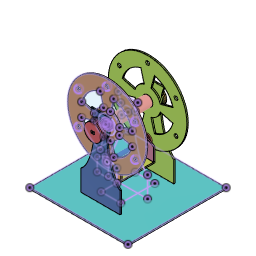
Ferris Wheel (Autodesk Fusion 360 design; units mm, degrees)
Autodesk Fusion 360 part; units mm, degrees
note: some values were not read from the file. Chosen so that the rebuilt part matches the saved one: where a step ends. Set by a fixed rule: which sketch regions a step uses.
sketch "01_base" plane through (0, 0, 0) normal (0, 0, 1) x (1, 0, 0) in component "05_centre_shaft"
  line L0 (75, -75) -> (-75, -75)
  line L1 (-75, -75) -> (-75, 75)
  line L2 (-75, 75) -> (75, 75)
  line L3 (75, 75) -> (75, -75)
  line L4 (75, -75) -> (-75, 75) construction
  line L5 (-75, -75) -> (75, 75) construction
  dimension "d1" = 150
  constraint horizontal L0
  constraint perpendicular L0 L1
  constraint parallel L0 L2
  constraint parallel L1 L3
  constraint coincident L4 origin
  constraint coincident L5 origin
  constraint equal L1 L2
  measures "d1" distance of L1.end L2.end
extrude "Extrude1" add sketch "01_base" along normal blind 2 makes body 1 in component "01_baseplate"
sketch "02_wheel" plane through (0, 0, 0) normal (0, 1, 0) x (1, 0, 0) in component "05_centre_shaft"
  circle A0 centre (0, -102) radius 60
  line L0 (-75, -2) -> (75, -2)
  line L1 (0, -1.75) -> (0, -22.5)
  circle A1 centre (0, -102) radius 40
  circle A2 centre (0, -152) radius 2.85
  line L2 (0, -162) -> (0, -142) construction
  circle A3 centre (43.3013, -127) radius 2.85
  circle A4 centre (43.3013, -77) radius 2.85
  circle A5 centre (0, -52) radius 2.85
  circle A6 centre (-43.3013, -77) radius 2.85
  circle A7 centre (-43.3013, -127) radius 2.85
  circle A8 centre (0, -102) radius 20
  line L3 (5.1764, -121.3185) -> (10.3528, -140.637)
  line L4 (-5.1764, -121.3185) -> (-10.3528, -140.637)
  line L5 (19.3185, -96.8236) -> (38.637, -91.6472)
  line L6 (19.3185, -107.1764) -> (38.637, -112.3528)
  line L7 (-5.1764, -82.6815) -> (-10.3528, -63.363)
  line L8 (5.1764, -82.6815) -> (10.3528, -63.363)
  line L9 (-19.3185, -107.1764) -> (-38.637, -112.3528)
  line L10 (-19.3185, -96.8236) -> (-38.637, -91.6472)
  circle A9 centre (0, -102) radius 7.95
  circle A10 centre (0, -52) radius 7
  line L11 (-3.5, -58.0622) -> (-15, -51.4226)
  line L12 (0, -42.7624) -> (0, -42)
  line L13 (0, -31.4226) -> (-15, -31.4226)
  line L14 (-15, -31.4226) -> (-15, -51.4226)
  line L15 (3.5, -58.0622) -> (15, -51.4226)
  line L16 (15, -31.4226) -> (15, -51.4226)
  line L17 (0, -31.4226) -> (15, -31.4226)
  point P0 (0, -152)
  dimension "d10" = 100
  dimension "d11" = 120
  dimension "d12" = -20
  dimension "d14" = 5.7
  dimension "d16" = 360
  dimension "d17" = -40
  dimension "d18" = 15
  dimension "d20" = 360
  dimension "d27" = 14
  dimension "d31" = 60
  dimension "d32" = 20
  dimension "d33" = 15
  dimension "d39" = 15.9
  constraint coincident A0.centre L1
  constraint coincident A0 L2.start
  constraint coincident A1 L2.end
  constraint coincident L1 L2.end
  constraint vertical L2
  constraint midpoint L2 P0
  constraint coincident P0 A2.centre
  constraint coincident A1 L3.end
  constraint coincident A8 L3.start
  constraint coincident A0.centre L3
  constraint symmetric L1 L3.end L4.end
  constraint symmetric L1 L3.start L4.start
  constraint concentric A0 A9
  constraint concentric A5 A10
  constraint tangent A10 L11
  constraint coincident A10 L11.start
  constraint vertical L12
  constraint horizontal L13
  constraint vertical L14
  constraint coincident L1 L13.start
  constraint coincident A0 L12.end
  constraint symmetric L1 L11.start L15.start
  constraint symmetric L1 L11.end L15.end
  constraint symmetric L1 L13.start L17.start
  constraint symmetric L1 L13.end L16.start
  measures "d10" distance of A0.centre L0
  measures "d11" diameter of A0
  measures "d14" diameter of A2
  measures "d18" angle of L1 L3
  measures "d27" diameter of A10
  measures "d31" angle of L1 L11
  measures "d32" distance of L11.end L13.end
  measures "d33" distance of L13.start L13.end
  measures "d39" diameter of A9
extrude "Extrude1'" add sketch "02_wheel" along normal blind 2 from surface at 30 separate body contours A0 A10 L11 L14 L15 L16 | A0 A10 L11 L14 L15 L16 | A10 | A1 A8 L5 L6 | A1 A8 L7 L8 | A8 | A1 A8 L3 L4 | A1 A8 L9 L10 makes body 2 in component "02_wheel"
mirror "MirrorComponent1" about plane through (0, 0, 0) normal (0, 0, 1) of bodies 2 makes body 3 in component "02_wheel(Mirror)"
extrude "Extrude1''" add sketch "02_wheel" along normal mid plane 75 separate body contours A5 makes body 4 in component "03_shaftouter"
extrude "Extrude1'''" add sketch "02_wheel" against normal blind 2 from surface at -32 separate body contours A10 makes body 5 in component "04_washer"
mirror "MirrorComponent2" about plane through (0, 0, 0) normal (0, 0, 1) of bodies 5 makes body 6 in component "04_washer(Mirror)"
extrude "Extrude1''''" add sketch "02_wheel" along normal blind 2 from surface at 24 separate body contours A0 A10 L11 L14 L15 L16 | A0 L13 L14 L16 L17 | A10 picked at (10.5828, -48.0695) makes body 7 in component "05_seat_side"
mirror "MirrorComponent3" about plane through (0, 0, 0) normal (0, 0, 1) of bodies 7 makes body 8 in component "05_seat_side(Mirror)"
sketch "03_seatbase" plane through (0, 0, 31.4226) normal (0, 0, -1) x (1, 0, 0) in component "05_centre_shaft"
  line L0 (-15, 24) -> (15, 24)
  line L1 (15, 24) -> (15, 26)
  line L2 (15, 26) -> (-15, 26)
  line L3 (-15, 26) -> (-15, 24)
  line L4 (15, -24) -> (15, -26)
  line L5 (3.5, -24) -> (15, -24)
  line L6 (3.5, -26) -> (15, -26)
  line L7 (-3.5, -24) -> (3.5, -24)
  line L8 (-3.5, -26) -> (3.5, -26)
  line L9 (-3.5, -24) -> (-15, -24)
  line L10 (-15, -26) -> (-3.5, -26)
  line L11 (-15, -24) -> (-15, -26)
  line L12 (15, 24) -> (15, 26)
  line L13 (3.5, 24) -> (15, 24)
  line L14 (3.5, 26) -> (15, 26)
  line L15 (-3.5, 24) -> (3.5, 24)
  line L16 (-3.5, 26) -> (3.5, 26)
  line L17 (-3.5, 24) -> (-15, 24)
  line L18 (-15, 24) -> (-15, 26)
  line L19 (-15, 26) -> (-3.5, 26)
  line L20 (-15, -26) -> (15, -26)
  line L21 (15, -26) -> (15, 26)
  line L22 (15, 26) -> (-15, 26)
  line L23 (-15, 26) -> (-15, -26)
  constraint horizontal L20
  constraint vertical L21
  constraint horizontal L22
  constraint vertical L23
  constraint coincident L1.end L2.start
  constraint coincident L10.start L11.end
extrude "Extrude1'''''" add sketch "03_seatbase" along normal blind 2 separate body makes body 9 in component "06_seat_bottom"
mirror "MirrorComponent4" about plane through (0, 0, 0) normal (0, 0, 1) of bodies 5 makes body 10 in component "04_washer(Mirror) (1)"
extrude "Extrude1''''''" add sketch "02_wheel" along normal blind 46 and the other way blind 46 separate body contours A9 makes body 11
sketch "test" plane through (0, 0, 0) normal (1, 0, 0) x (0, 1, 0) in component "05_centre_shaft"
  line L0 (-46, 102) -> (-46, 94.05)
  line L1 (-46, 109.95) -> (-46, 102)
  line L2 (46, 102) -> (46, 109.95)
  line L3 (46, 94.05) -> (46, 102)
  line L4 (-46, 94.05) -> (46, 94.05)
  line L5 (-46, 109.95) -> (46, 109.95)
  line L6 (-37.5, 52) -> (-37.5, 49.15)
  line L7 (-37.5, 54.85) -> (-37.5, 52)
  line L8 (37.5, 52) -> (37.5, 54.85)
  line L9 (37.5, 49.15) -> (37.5, 52)
  line L10 (-37.5, 49.15) -> (37.5, 49.15)
  line L11 (-37.5, 54.85) -> (37.5, 54.85)
  line L12 (38, 52) -> (38, 45)
  line L13 (38, 59) -> (38, 52)
  line L14 (36, 52) -> (36, 59)
  line L15 (36, 45) -> (36, 52)
  line L16 (38, 59) -> (36, 59)
  line L17 (38, 45) -> (36, 45)
  line L18 (46, 94.05) -> (46, 37.499) construction
  line L19 (38, 59) -> (46, 59)
  line L20 (37.5, 54.85) -> (38, 54.85)
  dimension "d44" = 8
  dimension "d45" = 0.5
  constraint coincident L3.start L4.end
  constraint perpendicular L17 L18
  constraint coincident L13.start L16.start
  constraint coincident L18 L19.end
  constraint perpendicular L18 L19
  constraint coincident L8.end L11.end
  constraint coincident L13 L20.end
  constraint perpendicular L13 L20
  measures "d44" distance of L13.start L19.end
  measures "d45" distance of L8.end L20.end
sketch "04_sidewalls" plane through (0, 46, 0) normal (0, 1, 0) x (-1, 0, 0) in component "05_centre_shaft"
  circle A0 centre (0, 102) radius 7.95
  circle A1 centre (0, 102) radius 7.95
  circle A2 centre (0, 102) radius 7.95
  circle A3 centre (0, 102) radius 12.95
  line L0 (-75, 2) -> (75, 2)
  line L1 (30, 2) -> (30, 122)
  line L2 (30, 2) -> (0, 2)
  line L3 (30, 122) -> (0, 122)
  line L4 (0, 1.75) -> (0, 22.5)
  line L5 (-30, 122) -> (0, 122)
  line L6 (-30, 2) -> (-30, 122)
  line L7 (-30, 2) -> (0, 2)
  spline S0 degree 5 poles (-15, 122) (-14.5292, 120.9084) (-13.6391, 118.6874) (-12.4585, 115.2425) (-11.1956, 110.4208) (-10.1478, 104.0108) (-9.6434, 97.2297) (-9.6878, 90.1157) (-10.2717, 82.7465) (-11.3574, 75.2596) (-12.8813, 67.8454) (-14.7677, 60.7196) (-16.9369, 54.1021) (-19.3146, 48.1926) (-21.8388, 43.1481) (-24.4697, 39.0478) (-26.6431, 36.5384) (-28.3081, 35.0867) (-29.4335, 34.3087) (-30, 33.9672) knots 0 0 0 0 0 0 0.066667 0.133333 0.2 0.266667 0.333333 0.4 0.466667 0.533333 0.6 0.666667 0.733333 0.8 0.866667 0.933333 1 1 1 1 1 1
  spline S1 degree 5 poles (15, 122) (14.5292, 120.9084) (13.6391, 118.6874) (12.4585, 115.2425) (11.1956, 110.4208) (10.1478, 104.0108) (9.6434, 97.2297) (9.6878, 90.1157) (10.2717, 82.7465) (11.3574, 75.2596) (12.8813, 67.8454) (14.7677, 60.7196) (16.9369, 54.1021) (19.3146, 48.1926) (21.8388, 43.1481) (24.4697, 39.0478) (26.6431, 36.5384) (28.3081, 35.0867) (29.4335, 34.3087) (30, 33.9672) knots 0 0 0 0 0 0 0.066667 0.133333 0.2 0.266667 0.333333 0.4 0.466667 0.533333 0.6 0.666667 0.733333 0.8 0.866667 0.933333 1 1 1 1 1 1
  line L8 (-18.4043, 129.8933) -> (-11.5957, 114.1067)
  line L9 (-24.0201, 37.5722) -> (-35.9799, 30.3621)
  line L10 (18.4043, 129.8933) -> (11.5957, 114.1067)
  line L11 (24.0201, 37.5722) -> (35.9799, 30.3621)
  line L12 (-2.475, 100.205) -> (-2.475, 103.795) construction
  line L13 (2.475, 103.795) -> (2.475, 100.205) construction
  arc A4 (-2.512, 103.6391) -> (-2.512, 100.3609) centre (4.7378, 102) ccw
  line L14 (2.3169, 100.205) -> (-2.3169, 100.205)
  line L15 (-2.3169, 103.795) -> (2.3169, 103.795)
  line L16 (-2.695, 102) -> (2.695, 102) construction
  arc A5 (-2.3169, 103.795) -> (-2.512, 103.6391) centre (-2.3169, 103.595) ccw
  arc A6 (2.512, 103.6391) -> (2.3169, 103.795) centre (2.3169, 103.595) ccw
  arc A7 (-2.512, 100.3609) -> (-2.3169, 100.205) centre (-2.3169, 100.405) ccw
  arc A8 (2.3169, 100.205) -> (2.512, 100.3609) centre (2.3169, 100.405) ccw
  arc A9 (2.512, 100.3609) -> (2.512, 103.6391) centre (-4.7378, 102) ccw
  point P0 (0, 94.05)
  point P1 (-15, 122)
  point P2 (-30, 33.9672)
  point P3 (-20, 47)
  point P4 (-10, 87)
  point P5 (-10, 87)
  point P6 (-20, 47)
  point P7 (10, 87)
  point P8 (20, 47)
  point P9 (0, 102)
  point P10 (0, 102)
  point P11 (0, 102)
  dimension "d48" = 15.9
  dimension "d49" = 5
  dimension "d52" = 120
  dimension "d53" = 30
  dimension "d54" = 20
  dimension "d58" = 20
  dimension "d59" = 35
  dimension "d60" = 10
  dimension "d61" = 75
  dimension "d64" = 4.95
  dimension "d21" = 3.59
  dimension "d66" = 5.39
  dimension "d67" = 0.2
  dimension "d68" = 0.2
  dimension "d69" = 0.2
  dimension "d70" = 0.2
  constraint concentric A1 A2
  constraint coincident A2 P0
  constraint concentric A2 A3
  constraint coincident L0 L1.start
  constraint perpendicular L0 L1
  constraint midpoint L0 L2.end
  constraint perpendicular L1 L3
  constraint coincident L3.end L4
  constraint symmetric L1.start L4 L6.start
  constraint symmetric L1.end L4 L5.start
  constraint symmetric L2.end L4 L7.end
  constraint symmetric L3.end L4 L5.end
  constraint midpoint L5 P1
  constraint coincident L6 P2
  constraint coincident P1 S0.start
  constraint coincident P5 P4
  constraint coincident P6 P3
  constraint coincident P2 S0.end
  constraint midpoint P1 L8
  constraint midpoint P2 L9
  constraint symmetric L4 P1 S1.start
  constraint symmetric L4 P5 P7
  constraint symmetric L4 P6 P8
  constraint symmetric L4 P2 S1.end
  constraint symmetric L4 L8.start L10.start
  constraint symmetric L4 L8.end L10.end
  constraint symmetric L4 L9.start L11.start
  constraint symmetric L4 L9.end L11.end
  constraint coincident P11 P10
  constraint horizontal L15
  constraint vertical L13
  constraint horizontal L14
  constraint vertical L12
  constraint horizontal L16
  constraint midpoint P11 L16
  constraint coincident L16.end A9
  constraint tangent L14 A7
  constraint tangent A4 A7
  constraint coincident L13.end L14
  constraint coincident L13.end A9
  constraint tangent L14 A8
  constraint tangent A8 A9
  constraint tangent L15 A5
  constraint tangent A4 A5
  constraint coincident L13.start L15
  constraint coincident L13.start A9
  constraint tangent L15 A6
  constraint tangent A6 A9
  measures "d48" diameter of A2
  measures "d49" distance of A2 A3
  measures "d52" distance of L1.start L1.end
  measures "d53" distance of origin L1
  measures "d54" distance of P10 L3.end
  measures "d58" distance of L6 P5
  measures "d59" vertical distance of L5.start P5
  measures "d60" distance of L6 P6
  measures "d61" distance of L5 P6
  measures "d64" distance of L13.start L12.end
  measures "d21" distance of L13.end L13.start
  measures "d66" distance of L16.end L16.start
  measures "d67" radius of A7
  measures "d68" radius of A8
  measures "d69" radius of A5
  measures "d70" radius of A6
extrude "Extrude1'''''''" add sketch "04_sidewalls" against normal blind 2 separate body contours A3 S1 | A3 S0 S1 | A3 S0 makes body 12 in component "06_centrestopper"
mirror "MirrorComponent5" about plane through (0, 0, 0) normal (0, 0, 1) of bodies 12 makes body 13 in component "06_centrestopper(Mirror)"
extrude "Extrude1''''''''" add sketch "04_sidewalls" against normal blind 2 from surface at -4 separate body contours A3 S1 | A3 L1 L3 S1 | A3 S0 S1 | A3 L3 L5 S0 S1 | A3 L0 L1 L2 L6 L7 S0 S1 | A3 S0 | A3 L5 L6 S0 makes body 14 in component "07_sidesupport"
mirror "MirrorComponent6" about plane through (0, 0, 0) normal (0, 0, 1) of bodies 14 makes body 15 in component "07_sidesupport(Mirror)"
extrude "Extrude2" cut sketch "04_sidewalls" along normal up to far side of body 14 contours A3 L1 L3 S1 | A3 L5 L6 S0 bodies 14 in component "07_sidesupport"
mirror "MirrorComponent7" about plane through (0, 0, 0) normal (0, 0, 1) of bodies 14 makes body 16 in component "07_sidesupport(Mirror) (1)"
extrude "Extrude1'''''''''" add sketch "04_sidewalls" against normal blind 2 from surface at -92 separate body contours A0 A1 A2 | A3 S1 | A3 S0 S1 | A3 S0 makes body 17 in component "08_motorslots"
sketch "lsr_horiz" plane through (0, 0, 2) normal (0, 0, 1) x (-1, 0, 0) in component "05_centre_shaft"
  line L0 (-75, -75) -> (75, -75)
  line L1 (75, -75) -> (75, 75)
  line L2 (75, 75) -> (-75, 75)
  line L3 (-75, 75) -> (-75, -75)
  line L4 (-75, -75) -> (-75, 75)
  line L5 (-75, 75) -> (75, 75)
  line L6 (75, 75) -> (75, -75)
  line L7 (75, -75) -> (-75, -75)
  line L8 (-15, 26) -> (15, 26)
  line L9 (-15, -26) -> (-15, 26)
  line L10 (15, -26) -> (-15, -26)
  line L11 (15, 26) -> (15, -26)
sketch "lsr_side_support" plane through (0, 0, 0) normal (0, 1, 0) x (1, 0, 0) in component "05_centre_shaft"
  arc A0 (11.0238, -108.7955) -> (9.7348, -93.4598) centre (0, -102) ccw
  spline S0 degree 3 poles (9.7348, -93.4598) (9.8417, -79.8722) (12.9149, -66.274) (17.8361, -51.6824) (20.0138, -46.3543) (23.7371, -40.266) (24.9309, -38.5784) (27.3687, -35.9118) (28.6123, -34.8037) (30, -33.9672) knots 0 0 0 0 4.076399 4.076399 6.121304 6.121304 6.912718 6.912718 7.556341 7.556341 7.556341 7.556341
  spline S1 degree 3 poles (15, -122) (14.1053, -119.9256) (13.3358, -117.8008) (12.0056, -113.3885) (11.4563, -111.1043) (11.0238, -108.7955) knots 0 0 0 0 0.677729 0.677729 1.382168 1.382168 1.382168 1.382168
  spline S2 degree 3 poles (-11.0238, -108.7955) (-11.4563, -111.1043) (-12.0056, -113.3885) (-13.3358, -117.8008) (-14.1053, -119.9256) (-15, -122) knots 0 0 0 0 0.704703 0.704703 1.382687 1.382687 1.382687 1.382687
  spline S3 degree 3 poles (-30, -33.9672) (-28.4163, -34.9219) (-27.0166, -36.2325) (-23.3261, -40.5136) (-21.2804, -44.2153) (-16.8467, -53.8264) (-14.4224, -61.4231) (-11.4968, -74.4671) (-9.8139, -83.4081) (-9.7348, -93.4598) knots 0 0 0 0 0.554769 0.554769 1.695754 1.695754 3.739955 3.739955 5.150418 5.150418 5.150418 5.150418
  arc A1 (-9.7348, -93.4598) -> (-11.0238, -108.7955) centre (0, -102) ccw
  circle A2 centre (0, -102) radius 7.95
  line L0 (-15, -122) -> (15, -122)
  line L1 (-30, -2) -> (-30, -33.9672)
  line L2 (30, -2) -> (-30, -2)
  line L3 (30, -33.9672) -> (30, -2)
sketch "lsr_washer" plane through (0, -32, 0) normal (0, -1, 0) x (1, 0, 0) in component "05_centre_shaft"
  line L0 (-5.1764, 82.6815) -> (-10.3528, 63.363)
  arc A0 (-38.637, 91.6472) -> (-10.3528, 63.363) centre (0, 102) ccw
  line L1 (-38.637, 91.6472) -> (-19.3185, 96.8236)
  arc A1 (-19.3185, 96.8236) -> (-5.1764, 82.6815) centre (0, 102) ccw
  circle A2 centre (0, 102) radius 7.95
  circle A3 centre (-43.3013, 127) radius 2.85
  circle A4 centre (-43.3013, 77) radius 2.85
  circle A5 centre (0, 52) radius 2.85
  circle A6 centre (0, 152) radius 2.85
  circle A7 centre (43.3013, 127) radius 2.85
  line L2 (19.3185, 96.8236) -> (38.637, 91.6472)
  arc A8 (10.3528, 63.363) -> (38.637, 91.6472) centre (0, 102) ccw
  line L3 (10.3528, 63.363) -> (5.1764, 82.6815)
  arc A9 (5.1764, 82.6815) -> (19.3185, 96.8236) centre (0, 102) ccw
  arc A10 (-5.1764, 121.3185) -> (-19.3185, 107.1764) centre (0, 102) ccw
  line L4 (-19.3185, 107.1764) -> (-38.637, 112.3528)
  arc A11 (-10.3528, 140.637) -> (-38.637, 112.3528) centre (0, 102) ccw
  line L5 (-10.3528, 140.637) -> (-5.1764, 121.3185)
  circle A12 centre (43.3013, 77) radius 2.85
  line L6 (5.1764, 121.3185) -> (10.3528, 140.637)
  arc A13 (38.637, 112.3528) -> (10.3528, 140.637) centre (0, 102) ccw
  line L7 (38.637, 112.3528) -> (19.3185, 107.1764)
  arc A14 (19.3185, 107.1764) -> (5.1764, 121.3185) centre (0, 102) ccw
  circle A15 centre (0, 102) radius 60
  circle A16 centre (0, 102) radius 7.95
  circle A17 centre (0, 102) radius 12.95
  circle A18 centre (0, 52) radius 2.85
  circle A19 centre (0, 52) radius 7
sketch "lsr_motor_support" plane through (0, -32, 0) normal (0, -1, 0) x (1, 0, 0) in component "05_centre_shaft"
  arc A0 (2.3169, 100.205) -> (2.512, 100.3609) centre (2.3169, 100.405) ccw
  arc A1 (2.512, 100.3609) -> (2.512, 103.6391) centre (-4.7378, 102) ccw
  arc A2 (2.512, 103.6391) -> (2.3169, 103.795) centre (2.3169, 103.595) ccw
  line L0 (2.3169, 103.795) -> (-2.3169, 103.795)
  arc A3 (-2.3169, 103.795) -> (-2.512, 103.6391) centre (-2.3169, 103.595) ccw
  arc A4 (-2.512, 103.6391) -> (-2.512, 100.3609) centre (4.7378, 102) ccw
  arc A5 (-2.512, 100.3609) -> (-2.3169, 100.205) centre (-2.3169, 100.405) ccw
  line L1 (-2.3169, 100.205) -> (2.3169, 100.205)
  circle A6 centre (0, 102) radius 12.95
sketch "lsr_wheel" plane through (0, -32, 0) normal (0, -1, 0) x (1, 0, 0) in component "05_centre_shaft"
  arc A0 (38.637, 112.3528) -> (10.3528, 140.637) centre (0, 102) ccw
  line L0 (19.3185, 107.1764) -> (38.637, 112.3528)
  arc A1 (19.3185, 107.1764) -> (5.1764, 121.3185) centre (0, 102) ccw
  line L1 (10.3528, 140.637) -> (5.1764, 121.3185)
  circle A2 centre (43.3013, 77) radius 2.85
  line L2 (-38.637, 112.3528) -> (-19.3185, 107.1764)
  arc A3 (-10.3528, 140.637) -> (-38.637, 112.3528) centre (0, 102) ccw
  line L3 (-5.1764, 121.3185) -> (-10.3528, 140.637)
  arc A4 (-5.1764, 121.3185) -> (-19.3185, 107.1764) centre (0, 102) ccw
  arc A5 (10.3528, 63.363) -> (38.637, 91.6472) centre (0, 102) ccw
  line L4 (5.1764, 82.6815) -> (10.3528, 63.363)
  arc A6 (5.1764, 82.6815) -> (19.3185, 96.8236) centre (0, 102) ccw
  line L5 (38.637, 91.6472) -> (19.3185, 96.8236)
  circle A7 centre (43.3013, 127) radius 2.85
  circle A8 centre (0, 152) radius 2.85
  circle A9 centre (0, 52) radius 2.85
  circle A10 centre (-43.3013, 77) radius 2.85
  circle A11 centre (-43.3013, 127) radius 2.85
  circle A12 centre (0, 102) radius 7.95
  arc A13 (-38.637, 91.6472) -> (-10.3528, 63.363) centre (0, 102) ccw
  line L6 (-19.3185, 96.8236) -> (-38.637, 91.6472)
  arc A14 (-19.3185, 96.8236) -> (-5.1764, 82.6815) centre (0, 102) ccw
  line L7 (-10.3528, 63.363) -> (-5.1764, 82.6815)
  circle A15 centre (0, 102) radius 60
sketch "lsr_swing_side" plane through (0, -32, 0) normal (0, -1, 0) x (1, 0, 0) in component "05_centre_shaft"
  circle A0 centre (0, 52) radius 2.85
  line L0 (-15, 31.4226) -> (15, 31.4226)
  line L1 (15, 31.4226) -> (15, 51.4226)
  line L2 (3.5, 58.0622) -> (15, 51.4226)
  arc A1 (3.5, 58.0622) -> (-3.5, 58.0622) centre (0, 52) ccw
  line L3 (-3.5, 58.0622) -> (-15, 51.4226)
  line L4 (-15, 31.4226) -> (-15, 51.4226)
component "01_baseplate" placed x (1, 0, 0) y (0, 1, 0) z (0, 0, 1) at (0, 0, 0)
component "02_wheel" placed x (1, 0, 0) y (0, 1, 0) z (0, 0, 1) at (0, 0, 0)
component "03_shaftouter" placed x (1, 0, 0) y (0, 1, 0) z (0, 0, 1) at (0, 0, 0)
component "04_washer" placed x (1, 0, 0) y (0, 1, 0) z (0, 0, 1) at (0, 0, 0)
component "04_washer" placed x (1, 0, 0) y (0, 1, 0) z (0, 0, 1) at (0, -2, 0)
component "04_washer" placed x (1, 0, 0) y (0, 1, 0) z (0, 0, 1) at (0, -4, 0)
component "05_seat_side" placed x (1, 0, 0) y (0, 1, 0) z (0, 0, 1) at (0, 0, 0)
component "06_seat_bottom" placed x (1, 0, 0) y (0, 1, 0) z (0, 0, 1) at (0, 0, 0)
component "04_washer" placed x (1, 0, 0) y (0, 1, 0) z (0, 0, 1) at (0, 62, 0)
component "04_washer" placed x (1, 0, 0) y (0, 1, 0) z (0, 0, 1) at (0, 60, 0)
component "02_wheel(Mirror)" placed x (1, 0, 0) y (0, -1, 0) z (0, 0, -1) at (0, 0, 0)
component "04_washer(Mirror)" placed x (1, 0, 0) y (0, -1, 0) z (0, 0, -1) at (0, 0, 0)
component "04_washer(Mirror)" placed x (1, 0, 0) y (0, -1, 0) z (0, 0, -1) at (0, 2, 0)
component "04_washer(Mirror)" placed x (1, 0, 0) y (0, -1, 0) z (0, 0, -1) at (0, 4, 0)
component "05_seat_side(Mirror)" placed x (1, 0, 0) y (0, -1, 0) z (0, 0, -1) at (0, 0, 0)
component "04_washer(Mirror) (1)" placed x (1, 0, 0) y (0, -1, 0) z (0, 0, -1) at (0, -62, 0)
component "04_washer(Mirror) (1)" placed x (1, 0, 0) y (0, -1, 0) z (0, 0, -1) at (0, -60, 0)
component "05_centre_shaft" placed x (1, 0, 0) y (0, 1, 0) z (0, 0, 1) at (0, 0, 0)
component "06_centrestopper" placed x (1, 0, 0) y (0, 1, 0) z (0, 0, 1) at (0, 0, 0)
component "06_centrestopper" placed x (1, 0, 0) y (0, 1, 0) z (0, 0, 1) at (0, -2, 0)
component "07_sidesupport" placed x (1, 0, 0) y (0, 1, 0) z (0, 0, 1) at (0, 0, 0)
component "06_centrestopper(Mirror)" placed x (1, 0, 0) y (0, -1, 0) z (0, 0, -1) at (0, 0, 0)
component "06_centrestopper(Mirror)" placed x (1, 0, 0) y (0, -1, 0) z (0, 0, -1) at (0, 2, 0)
component "07_sidesupport(Mirror) (1)" placed x (1, 0, 0) y (0, -1, 0) z (0, 0, -1) at (0, 0, 0)
component "08_motorslots" placed x (1, 0, 0) y (0, 1, 0) z (0, 0, 1) at (0, 0, 0)
component "08_motorslots" placed x (1, 0, 0) y (0, 1, 0) z (0, 0, 1) at (0, -2, 0)
component "08_motorslots" placed x (1, 0, 0) y (0, 1, 0) z (0, 0, 1) at (0, -4, 0)
component "08_motorslots" placed x (1, 0, 0) y (0, 1, 0) z (0, 0, 1) at (0, -6, 0)
equation "d1 = board2mm"
equation "board2mm = 150 mm" comment "Dimension of 2 mm Board"
equation "thick_2 = 2 mm" comment "Board Thickness"
equation "thick_3 = 3 mm" comment "Board Thickness"
equation "d8 = thick_2"
equation "d10 = 60 mm + 40 mm"
equation "shaft_dia = 5.7 mm" comment "Edit as per req"
equation "d14 = shaft_dia"
equation "d23 = thick_2"
equation "d29 = -thick_2"
equation "d35 = thick_2"
equation "d37 = thick_2"
equation "d39 = center_shaft"
equation "center_shaft = 15.9 mm" comment "PVC Pipe Dia"
equation "d50 = -thick_2"
equation "d56 = -thick_2"
equation "d67 = crank_fillet"
equation "d68 = crank_fillet"
equation "d69 = crank_fillet"
equation "d70 = crank_fillet"
equation "d72 = -thick_2"
